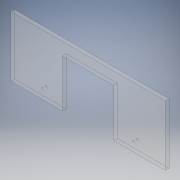
# Autodesk Inventor part: Front wall
Saved by Autodesk Inventor 2019 (Build 230136000, 136)
## iProperties
Created: 2018-08-29
Part Number: Front wall
Material: Polycarbonate, Clear
Document SubType Name: Modeling
Designer: kalakuntla1297
Density: 1.2 g/cm^3
Appearance: Polycarbonate - Clear
Author: kalakuntla1297
Autodesk Inventor part; units mm, degrees
ref_plane "YZ Plane" through (0, 0, 0) normal (1, 0, 0) x (0, 1, 0)
ref_plane "XZ Plane" through (0, 0, 0) normal (0, 1, 0) x (-1, 0, 0)
ref_plane "XY Plane" through (0, 0, 0) normal (0, 0, 1) x (1, 0, 0)
sketch "Sketch1" plane through (0, 0, 0) normal (0, 0, 1) x (1, 0, 0)
  line L0 (0, 0) -> (533.4, 0)
  line L1 (533.4, 0) -> (533.4, 208.28)
  line L2 (533.4, 208.28) -> (0, 208.28)
  line L3 (0, 208.28) -> (0, 0)
  dimension "d0" = 533.4
  dimension "d1" = 208.28
  constraints: 8 end point, 2 parallel, 1 horizontal, 1 perpendicular
  measures "d0" distance of L0.start L0.end
  measures "d1" distance of L0.end L1.end
extrude "Extrusion1" add sketch "Sketch1" along normal blind 12.7
sketch "Sketch2" plane through (0, 0, 12.7) normal (0, 0, 1) x (1, 0, 0)
  line L0 (0, 0) -> (533.4, 0) projected
  line L1 (355.6, 0) -> (177.8, 0)
  line L2 (177.8, 0) -> (177.8, 165.1)
  line L3 (177.8, 165.1) -> (355.6, 165.1)
  line L4 (355.6, 165.1) -> (355.6, 0)
  line L5 (533.4, 0) -> (533.4, 208.28) projected
  line L6 (0, 208.28) -> (0, 0) projected
  dimension "d4" = 165.1
  dimension "d5" = 177.8
  dimension "d6" = 177.8
  constraints: 8 end point, 2 parallel, 1 horizontal, 1 perpendicular, 1 point on line
  measures "d4" distance of L3.end L1.start
  measures "d5" distance between parallel lines of L4 L5
  measures "d6" distance between parallel lines of L6 L2
extrude "Extrusion2" cut sketch "Sketch2" against normal blind 12.7
sketch "Sketch3" plane through (0, 0, 12.7) normal (0, 0, 1) x (1, 0, 0)
  circle A0 centre (423.926, 31.75) radius 4.1656
  line L0 (533.4, 0) -> (533.4, 208.28) projected
  circle A1 centre (109.474, 31.75) radius 4.1656
  line L1 (0, 208.28) -> (0, 0) projected
  line L2 (0, 0) -> (177.8, 0) projected
  line L3 (355.6, 0) -> (533.4, 0) projected
  dimension "d9" = 109.474
  dimension "d10" = 8.3312
  dimension "d11" = 8.3312
  dimension "d12" = 109.474
  dimension "d13" = 31.75
  dimension "d14" = 31.75
  constraints: 2 centre point
  measures "d9" distance from line of L0 A0.centre
  measures "d10" diameter of A1
  measures "d11" diameter of A0
  measures "d12" distance from line of L1 A1.centre
  measures "d13" distance from line of L2 A1.centre
  measures "d14" distance from line of L3 A0.centre
extrude "Extrusion3" cut sketch "Sketch3" against normal blind 25.4
body "Solid1"
